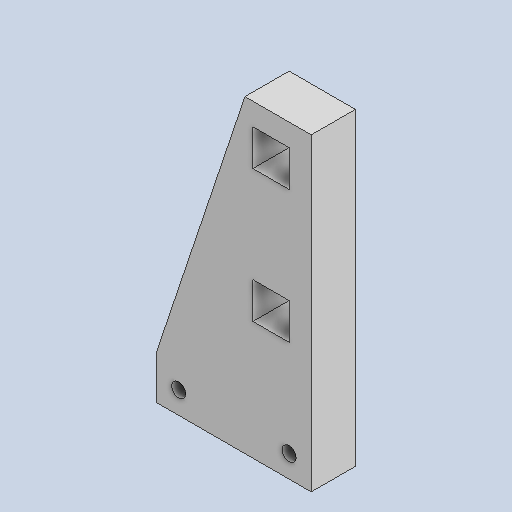
# Autodesk Inventor part: Soporte lateral
Saved by Autodesk Inventor 2024 (Build 280153000, 153)
## iProperties
Created: 2025-03-01
Part Number: Soporte lateral
Material: Genérico
Document SubType Name: Modeling
Designer: sergi
Density: 1 g/cm^3
Appearance: Valor por defecto
Author: sergi
Autodesk Inventor part; units mm, degrees
ref_plane "YZ Plane" through (0, 0, 0) normal (1, 0, 0) x (0, 1, 0)
ref_plane "XZ Plane" through (0, 0, 0) normal (0, 1, 0) x (-1, 0, 0)
ref_plane "XY Plane" through (0, 0, 0) normal (0, 0, 1) x (1, 0, 0)
sketch "Boceto1" plane through (0, 0, 0) normal (0, 0, 1) x (1, 0, 0)
  line L0 (0, 0) -> (105, 0)
  line L1 (105, 0) -> (105, 60)
  line L2 (105, 60) -> (0, 0)
  line L3 (105, 60) -> (90, 60)
  line L4 (90, 60) -> (0, 0)
  line L5 (0, 0) -> (70, 0)
  line L6 (70, 0) -> (90, 60)
  dimension "d0" = 105
  dimension "d1" = 60
  dimension "d4" = 15
  dimension "d10" = 70
  constraints: 14 end point, 2 horizontal, 1 perpendicular, 1 point on line
  measures "d0" distance of L0.start L0.end
  measures "d1" distance of L0.end L1.end
  measures "d4" distance of L1.end L3.end
  measures "d10" distance of L0.start L5.end
extrude "Extrusión1" add sketch "Boceto1" along normal blind 10 contours L6 L2 L1 L0 | L6 L3 L2
sketch "Boceto2" plane through (0, 0, 10) normal (0, 0, 1) x (1, 0, 0)
  line L0 (-12.3369, 16.82) -> (-7.4631, 16.82) projected
  line L1 (-3.8564, 16.82) -> (-7.4631, 16.82) projected
  line L2 (-3.8564, 16.82) -> (105, 16.82)
  line L3 (105, 0) -> (105, 60) projected
  line L4 (105, 60) -> (90, 60) projected
  line L5 (70, 0) -> (105, 0) projected
  line L6 (100, 5) -> (14.5727, 5)
  line L7 (91.7155, 55) -> (100, 55)
  line L8 (100, 16.82) -> (91.8, 16.82)
  line L9 (91.8, 16.82) -> (91.8, 25.02)
  line L10 (91.8, 25.02) -> (100, 25.02)
  line L11 (100, 25.02) -> (100, 16.82)
  line L12 (90, 60) -> (70, 0) projected
  line L13 (91.8, 55) -> (91.8, 46.8)
  line L14 (91.8, 46.8) -> (100, 46.8)
  line L15 (100, 46.8) -> (100, 55)
  line L16 (105, 60) -> (105, 55)
  line L17 (105, 60) -> (110, 60) construction
  line L18 (105, 55) -> (91.8, 55)
  point P0 (0, 0)
  point P1 (91.8, 55)
  dimension "d6" = 8.2
  dimension "d7" = 8.2
  dimension "d11" = 8.2
  dimension "d21" = 5
  dimension "d22" = 90
  constraints: 26 end point, 3 horizontal, 3 parallel, 3 perpendicular, 1 collinear, 1 point on line
  measures "d6" distance of L9.end L10.end
  measures "d7" distance of L8.end L9.end
  measures "d11" distance of L13.end L13.start
  measures "d21" distance of L3.end L16.end
  measures "d22" angle of L16 L17
extrude "Extrusión2" cut sketch "Boceto2" against normal through all contours L9 L10 L11 L2 | L7 L15 L14 L13
sketch "Boceto3" plane through (70, 0, 0) normal (0, -1, 0) x (1, 0, 0)
  line L0 (21.8, 10) -> (21.8, 0) projected
  line L1 (0, 10) -> (35, 10) projected
  line L2 (0, 0) -> (35, 0) projected
  line L3 (35, 0) -> (35, 10) projected
  line L4 (0, 10) -> (0, 0) projected
  point P0 (-70, 0)
extrude "Extrusión3" add sketch "Boceto3" along normal blind 10
sketch "Boceto4" plane through (0, 0, 10) normal (0, 0, 1) x (1, 0, 0)
  circle A0 centre (75, -5) radius 2.1 projected
  circle A1 centre (100, -5) radius 2.1 projected
  point P0 (0, 0)
hole "Agujero1" at (75, -5, 10) at (100, -5, 10) direction (0, 0, -1) diameter 3.2 depth 10
